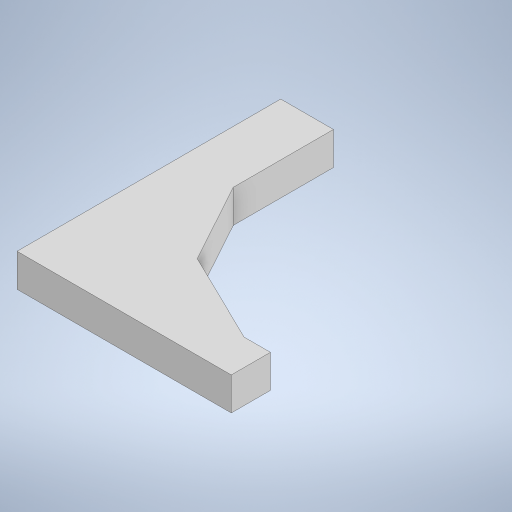
# Autodesk Inventor part: FlanecElement
Saved by Autodesk Inventor 2024 (Build 280153000, 153)
## iProperties
Created: 2023-11-20
Part Number: FlanecElement
Material: Generic
Document SubType Name: Modeling
Designer: KirikDK
Density: 1 g/cm^3
Appearance: Default
Author: KirikDK
Autodesk Inventor part; units mm, degrees
ref_plane "YZ Plane" through (0, 0, 0) normal (1, 0, 0) x (0, 1, 0)
ref_plane "XZ Plane" through (0, 0, 0) normal (0, 1, 0) x (-1, 0, 0)
ref_plane "XY Plane" through (0, 0, 0) normal (0, 0, 1) x (1, 0, 0)
sketch "Sketch1" plane through (0, 0, 0) normal (0, 1, 0) x (-1, 0, 0)
  line L0 (37, 70) -> (-28, 70)
  line L1 (-28, 70) -> (-28, -10)
  line L2 (-28, -10) -> (37, -10)
  line L3 (37, -10) -> (37, 70)
  circle A0 centre (-28, 6.4944) radius 52.237
  line L4 (21, -32) -> (21, 20.4)
  line L5 (21, 20.4) -> (-15, 86)
  line L6 (7.7078, 44.6213) -> (-20, 58.1152)
  line L7 (-20, 58.1152) -> (-28, 58.1152)
  point P0 (0, 0)
  point P1 (-28, 58.7314)
  point P2 (21.5645, -10)
  point P3 (3.7799, 47.9522)
  point P4 (21, -10)
  dimension "d0" = 65
  dimension "d1" = 80
  dimension "d5" = 16
  dimension "d6" = 52.4
  constraints: 16 end point, 3 point on line, 2 parallel, 2 perpendicular, 2 point on circle, 1 centre point, 1 horizontal, 1 vertical
  measures "d0" distance of L0.start L0.end
  measures "d1" distance of L2.end L0.start
  measures "d5" distance between parallel lines of L3 L4
  measures "d6" distance of L4.start L4.end
extrude "Extrusion1" add sketch "Sketch1" along normal blind 10 contours L3 L2 A0 L5 L0 | L5 A0 L1 L0 | L6 A0 | A0 L2 L4 L5 | A0 L7 L1
body "Solid1"
